# Autodesk Inventor part: LAN8710A_QFN32
Saved by Autodesk Inventor 2015 SP1 (Build 190203100, 203)
## iProperties
Created: 2015-06-25
Part Number: LAN8710A_QFN32
Material: Generic
Document SubType Name: Modeling
Designer: Patrick
Density: 1 g/cm^3
Appearance: QFN32, LAN8710A_QFN32
Author: Patrick
Autodesk Inventor part; units mm, degrees
ref_plane "YZ Plane" through (0, 0, 0) normal (1, 0, 0) x (0, 1, 0)
ref_plane "XZ Plane" through (0, 0, 0) normal (0, 1, 0) x (-1, 0, 0)
ref_plane "XY Plane" through (0, 0, 0) normal (0, 0, 1) x (1, 0, 0)
sketch "QFN32, LAN8710A_QFN32_127" plane through (0, 0, 0) normal (0, 0, 1) x (1, 0, 0)
  line L0 (-3.202, -3.925) -> (-3.202, 3.202)
  line L1 (-3.202, 3.202) -> (3.202, 3.202)
  line L2 (3.202, 3.202) -> (3.202, -3.925)
  line L3 (3.202, -3.925) -> (-3.202, -3.925)
  constraints: 8 end point
extrude "Extrusion1" add sketch "QFN32, LAN8710A_QFN32_127" along normal blind 1
body "Solid1"
